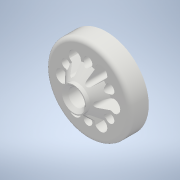
# Autodesk Inventor part: ОпорныйКаток2
Saved by Autodesk Inventor 2020 (Build 240168000, 168)
## iProperties
Created: 2021-03-04
Part Number: ОпорныйКаток2
Material: Пластик АБС
Document SubType Name: Modeling
Designer: I_Love_U_Bogdan
Density: 1.06 g/cm^3
Appearance: Гладкий — белый
Author: I_Love_U_Bogdan
Autodesk Inventor part; units mm, degrees
ref_plane "YZ Plane" through (0, 0, 0) normal (1, 0, 0) x (0, 1, 0)
ref_plane "XZ Plane" through (0, 0, 0) normal (0, 1, 0) x (-1, 0, 0)
ref_plane "XY Plane" through (0, 0, 0) normal (0, 0, 1) x (1, 0, 0)
sketch "Эскиз1" plane through (0, 0, 0) normal (0, 0, 1) x (1, 0, 0)
  arc A0 (2.629995, 7.384738) -> (5.080374, 5.970011) centre (4.104457, 7.109128) ccw
  line L0 (2.629995, 7.384738) -> (3.506381, 12.073229)
  arc A1 (8.702533, 9.073229) -> (3.506381, 12.073229) centre (6.104457, 10.573229) ccw
  line L1 (8.702533, 9.073229) -> (5.080374, 5.970011)
  circle A2 centre (10.392305, -6) radius 2
  circle A3 centre (-10.392305, -6) radius 2
  line L2 (-12.208913, 3) -> (-7.710368, 1.414727)
  arc A4 (-7.710368, -1.414727) -> (-7.710368, 1.414727) centre (-8.208913, 0) ccw
  line L3 (-7.710368, -1.414727) -> (-12.208913, -3)
  arc A5 (-12.208913, 3) -> (-12.208913, -3) centre (-12.208913, 0) ccw
  arc A6 (3.506381, -12.073229) -> (8.702533, -9.073229) centre (6.104457, -10.573229) ccw
  line L4 (3.506381, -12.073229) -> (2.629995, -7.384738)
  arc A7 (5.080374, -5.970011) -> (2.629995, -7.384738) centre (4.104457, -7.109128) ccw
  line L5 (5.080374, -5.970011) -> (8.702533, -9.073229)
  circle A8 centre (0, 12) radius 2
  arc A9 (-5.080374, 5.970011) -> (-2.629995, 7.384738) centre (-4.104457, 7.109128) ccw
  line L6 (-5.080374, 5.970011) -> (-8.702533, 9.073229)
  arc A10 (-3.506381, 12.073229) -> (-8.702533, 9.073229) centre (-6.104457, 10.573229) ccw
  line L7 (-3.506381, 12.073229) -> (-2.629995, 7.384738)
  line L8 (12.208913, -3) -> (7.710368, -1.414727)
  arc A11 (7.710368, 1.414727) -> (7.710368, -1.414727) centre (8.208913, 0) ccw
  line L9 (7.710368, 1.414727) -> (12.208913, 3)
  arc A12 (12.208913, -3) -> (12.208913, 3) centre (12.208913, 0) ccw
  line L10 (-8.702533, -9.073229) -> (-5.080374, -5.970011)
  arc A13 (-2.629995, -7.384738) -> (-5.080374, -5.970011) centre (-4.104457, -7.109128) ccw
  line L11 (-2.629995, -7.384738) -> (-3.506381, -12.073229)
  arc A14 (-8.702533, -9.073229) -> (-3.506381, -12.073229) centre (-6.104457, -10.573229) ccw
  circle A15 centre (-10.392305, 6) radius 2
  circle A16 centre (0, -12) radius 2
  circle A17 centre (10.392305, 6) radius 2
  circle A18 centre (0, 0) radius 4
  circle A19 centre (0, 0) radius 20
extrude "Выдавливание1" add sketch "Эскиз1" along normal blind 8.7 contours A2 | A3 | A8 | A15 | A16 | A17 | A19
sketch "Эскиз2" plane through (0, 0, 0) normal (0, 0, -1) x (-1, 0, 0)
  circle A0 centre (10.392305, 6) radius 2
  circle A1 centre (10.392305, -6) radius 2
  circle A2 centre (0, -12) radius 2
  circle A3 centre (-10.392305, -6) radius 2
  circle A4 centre (-10.392305, 6) radius 2
  circle A5 centre (0, 12) radius 2
  circle A6 centre (0, 12) radius 2.05
  circle A7 centre (-10.392305, 6) radius 2.05
  circle A8 centre (-10.392305, -6) radius 2.05
  circle A9 centre (0, -12) radius 2.05
  circle A10 centre (10.392305, -6) radius 2.05
  circle A11 centre (10.392305, 6) radius 2.05
  point P0 (0, 0)
  dimension "d15" = 4.1
  dimension "d18" = 360
  constraints: 6 centre point, 1 coincident, 13 other
  measures "d15" diameter of A6
extrude "Выдавливание2" cut sketch "Эскиз2" against normal up to surface (8.7 mm away) contours A0 | A1 | A2 | A3 | A4 | A5 | A6 | A7 | A8 | A9 | A10 | A11
fillet "Сопряжение1" radius 2 1 edges at (-20, 0, 8.7)
sketch "Эскиз3" plane through (0, 0, 8.7) normal (0, 0, 1) x (1, 0, 0)
  circle A0 centre (0, 0) radius 6
  circle A1 centre (0, 0) radius 4 projected
  dimension "d5" = 2
  constraints: 1 centre point, 1 coincident
  measures "d5" radial gap between concentric circles of A1 A0
extrude "Выдавливание3" add sketch "Эскиз3" along normal blind 6.8
chamfer "Фаска1" distance 5 angle 45 1 edges at (-6, 0, 8.7)
chamfer "Фаска2" distance 1.5 angle 45 1 edges at (-4, 0, 15.5)
chamfer "Фаска3" distance 0.5 angle 45 1 edges at (-4, 0, 0)
chamfer "Фаска4" distance 0.5 angle 45 6 edges at (12.4423, -6, 0) (2.05, -12, 0) (-8.3423, -6, 0) (-8.3423, 6, 0) (2.05, 12, 0) (12.4423, 6, 0)
